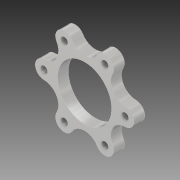
# Autodesk Inventor part: Standardized Plate Spacer
Saved by Autodesk Inventor 2022 (Build 260153000, 153)
## iProperties
Created: 2019-01-17
Part Number: Standardized Plate Spacer
Material: Aluminum 6061
Document SubType Name: Modeling
Designer: Max Boord
Density: 2.7 g/cm^3
Appearance: Aluminum - Dark
Mass: 15.3927 g
Surface Area: 42.1109 cm^2
Volume: 5.701 cm^3
Author: Max Boord
Autodesk Inventor part; units mm, degrees
ref_plane "YZ Plane" through (0, 0, 0) normal (1, 0, 0) x (0, 1, 0)
ref_plane "XZ Plane" through (0, 0, 0) normal (0, 1, 0) x (-1, 0, 0)
ref_plane "XY Plane" through (0, 0, 0) normal (0, 0, 1) x (1, 0, 0)
sketch "Sketch1" plane through (0, 0, 0) normal (0, 0, 1) x (1, 0, 0)
  circle A0 centre (0, 0) radius 19.05
  circle A1 centre (23.8125, 0) radius 2.0193
  arc A2 (23.8832, -5.1938) -> (23.8832, 5.1938) centre (23.8125, 0) ccw
  arc A3 (16.4978, 9.525) -> (23.8832, 5.1938) centre (24.001, 13.857) ccw
  arc A4 (23.8832, -5.1938) -> (16.4978, -9.525) centre (24.001, -13.857) ccw
  circle A5 centre (11.9063, 20.6222) radius 2.0193
  arc A6 (16.4396, 18.0865) -> (7.4436, 23.2803) centre (11.9063, 20.6222) ccw
  arc A7 (0, 19.05) -> (7.4436, 23.2803) centre (0, 27.714) ccw
  arc A8 (16.4396, 18.0865) -> (16.4978, 9.525) centre (24.001, 13.857) ccw
  circle A9 centre (-11.9062, 20.6222) radius 2.0193
  arc A10 (-7.4436, 23.2803) -> (-16.4396, 18.0865) centre (-11.9062, 20.6222) ccw
  arc A11 (-16.4978, 9.525) -> (-16.4396, 18.0865) centre (-24.001, 13.857) ccw
  arc A12 (-7.4436, 23.2803) -> (0, 19.05) centre (0, 27.714) ccw
  circle A13 centre (-23.8125, 0) radius 2.0193
  arc A14 (-23.8832, 5.1938) -> (-23.8832, -5.1938) centre (-23.8125, 0) ccw
  arc A15 (-16.4978, -9.525) -> (-23.8832, -5.1938) centre (-24.001, -13.857) ccw
  arc A16 (-23.8832, 5.1938) -> (-16.4978, 9.525) centre (-24.001, 13.857) ccw
  circle A17 centre (-11.9063, -20.6222) radius 2.0193
  arc A18 (-16.4396, -18.0865) -> (-7.4436, -23.2803) centre (-11.9063, -20.6222) ccw
  arc A19 (0, -19.05) -> (-7.4436, -23.2803) centre (0, -27.714) ccw
  arc A20 (-16.4396, -18.0865) -> (-16.4978, -9.525) centre (-24.001, -13.857) ccw
  circle A21 centre (11.9062, -20.6222) radius 2.0193
  arc A22 (7.4436, -23.2803) -> (16.4396, -18.0865) centre (11.9062, -20.6222) ccw
  arc A23 (16.4978, -9.525) -> (16.4396, -18.0865) centre (24.001, -13.857) ccw
  arc A24 (7.4436, -23.2803) -> (0, -19.05) centre (0, -27.714) ccw
  circle A25 centre (0, 0) radius 15.875
  dimension "d0" = 38.1
  dimension "d1" = 4.0386
  dimension "d2" = 3.175
  dimension "d3" = 23.8125
  dimension "d4" = 8.664
  dimension "d7" = 360
  dimension "d9" = 31.75
  constraints: 38 point on circle, 26 centre point, 4 tangent, 2 coincident, 1 equal radius, 1 horizontal alignment, 67 other
  measures "d0" diameter of A0
  measures "d1" diameter of A1
  measures "d2" radial gap between concentric circles of A1 A2
  measures "d3" distance of A1.centre point (0, 0)
  measures "d4" radius of A3
  measures "d9" diameter of A25
extrude "Extrusion1" add sketch "Sketch1" along normal blind 6.35 contours A0 | A0 A3 A2 A4
pattern_circular "Circular Pattern1" count 6 over 360 about axis through (0, 0, 0) along (0, 0, 1) of "Extrusion1"
body "Solid1"
